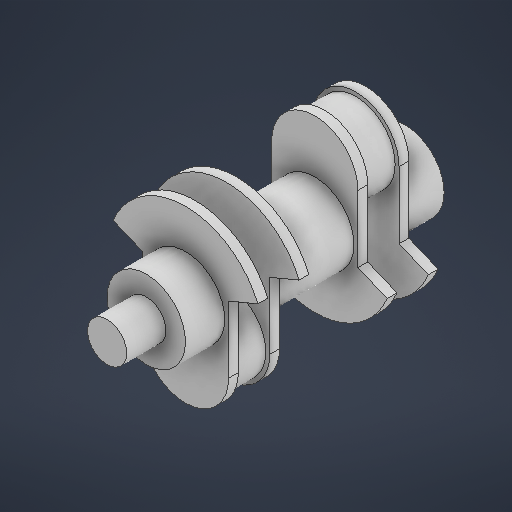
# Autodesk Inventor part: crankshaft
Saved by Autodesk Inventor 2026.1 (Build 301233020, 233B)
## iProperties
Created: 2025-12-11
Part Number: crankshaft
Material: Generic
Document SubType Name: Modeling
Designer: ender
Density: 1 g/cm^3
Appearance: Default
Author: ender
Autodesk Inventor part; units mm, degrees
ref_plane "YZ Plane" through (0, 0, 0) normal (1, 0, 0) x (0, 1, 0)
ref_plane "XZ Plane" through (0, 0, 0) normal (0, 1, 0) x (-1, 0, 0)
ref_plane "XY Plane" through (0, 0, 0) normal (0, 0, 1) x (1, 0, 0)
sketch "Sketch1" plane through (0, 0, 0) normal (0, 0, 1) x (1, 0, 0)
  circle A0 centre (0, 0) radius 25.4
  dimension "d0" = 50.8
  constraints: 1 centre point, 1 coincident
  measures "d0" diameter of A0
extrude "Extrusion1" add sketch "Sketch1" along normal blind 25.4
sketch "Sketch2" plane through (0, 0, 25.4) normal (0, 0, 1) x (1, 0, 0)
  arc A0 (27.94, 31.75) -> (-27.94, 31.75) centre (0, 31.75) ccw
  arc A1 (-46.9331, -19.4403) -> (46.9331, -19.4403) centre (0, 0) ccw
  line L0 (-27.94, 31.75) -> (-27.94, -11.5731)
  line L1 (-27.94, -11.5731) -> (-46.9331, -19.4403)
  line L2 (27.94, 31.75) -> (27.94, -11.5731)
  line L3 (27.94, -11.5731) -> (46.9331, -19.4403)
  circle A2 centre (0, 0) radius 25.4 projected
  dimension "d3" = 31.75
  dimension "d4" = 50.8
  dimension "d5" = 27.94
  dimension "d6" = 135
  constraints: 8 end point, 4 point on circle, 2 centre point, 2 coincident, 2 equal length, 2 point on line, 2 vertical, 1 tangent, 1 vertical alignment
  measures "d3" distance of A0.centre A2.centre
  measures "d4" radius of A1
  measures "d5" radius of A0
  measures "d6" angle of L3 L1
extrude "Extrusion2" add sketch "Sketch2" along normal blind 6.35 contours L2 L3 A1 L1 L0 A0 | A2
sketch "Sketch3" plane through (0, 0, 31.75) normal (0, 0, 1) x (1, 0, 0)
  circle A0 centre (0, 31.75) radius 25.4
  arc A1 (27.94, 31.75) -> (-27.94, 31.75) centre (0, 31.75) ccw projected
  point P0 (0, 0)
  dimension "d9" = 50.8
  constraints: 1 centre point, 1 concentric
  measures "d9" diameter of A0
extrude "Extrusion3" add sketch "Sketch3" along normal blind 20.32
pattern_linear "Rectangular Pattern1" count 2 spacing 26.67 along (0, 0, 1) of "Extrusion2"
sketch "Sketch4" plane through (0, 0, 58.42) normal (0, 0, 1) x (1, 0, 0)
  circle A0 centre (0, 0) radius 25.4
  dimension "d15" = 50.8
  constraints: 1 centre point, 1 coincident
  measures "d15" diameter of A0
extrude "Extrusion4" add sketch "Sketch4" along normal blind 50.8
sketch "Sketch5" plane through (0, 4.445, 109.22) normal (0, 0, 1) x (-1, 0, 0)
  arc A0 (27.94, 36.195) -> (-27.94, 36.195) centre (0, 36.195) ccw
  arc A1 (-46.9331, -14.9953) -> (46.9331, -14.9953) centre (0, 4.445) ccw
  line L0 (-27.94, 36.195) -> (-27.94, -7.1281)
  line L1 (-27.94, -7.1281) -> (-46.9331, -14.9953)
  line L2 (27.94, 36.195) -> (27.94, -7.1281)
  line L3 (27.94, -7.1281) -> (46.9331, -14.9953)
  circle A2 centre (0, 4.445) radius 25.4 projected
  point P0 (0, 4.445)
  dimension "d19" = 50.8
  dimension "d20" = 27.94
  dimension "d18" = 135
  dimension "d25" = 31.75
  constraints: 8 end point, 4 point on circle, 2 centre point, 2 coincident, 2 equal length, 2 point on line, 2 vertical, 1 concentric, 1 tangent, 1 vertical alignment
  measures "d19" radius of A1
  measures "d20" radius of A0
  measures "d18" angle of L3 L1
  measures "d25" distance of A2.centre A0.centre
extrude "Extrusion5" add sketch "Sketch5" along normal blind 6.35 contours L2 L3 A1 L1 L0 A0 | A2
sketch "Sketch6" plane through (0, 4.445, 115.57) normal (0, 0, 1) x (1, 0, 0)
  circle A0 centre (0, -36.195) radius 25.4
  arc A1 (-27.94, -36.195) -> (27.94, -36.195) centre (0, -36.195) ccw projected
  point P0 (0, -4.445)
  dimension "d26" = 50.8
  constraints: 1 centre point, 1 concentric
  measures "d26" diameter of A0
extrude "Extrusion6" add sketch "Sketch6" along normal blind 25.4
pattern_linear "Rectangular Pattern2" count 2 spacing 26.67 along (0, 0, 1) of "Extrusion5"
sketch "Sketch7" plane through (0, 0, 142.24) normal (0, 0, 1) x (1, 0, 0)
  circle A0 centre (0, 0) radius 25.4
  dimension "d32" = 50.8
  constraints: 1 centre point, 1 coincident
  measures "d32" diameter of A0
extrude "Extrusion7" add sketch "Sketch7" along normal blind 25.4
sketch "Sketch8" plane through (0, 0, 167.64) normal (0, 0, 1) x (1, 0, 0)
  circle A0 centre (0, 0) radius 12.7
  dimension "d35" = 25.4
  constraints: 1 centre point, 1 coincident
  measures "d35" diameter of A0
extrude "Extrusion8" add sketch "Sketch8" along normal blind 25.4
body "Solid1"
